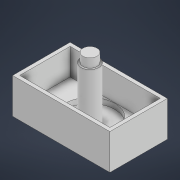
# Autodesk Inventor part: Servoverbindung_Konzept
Saved by Autodesk Inventor 2021 (Build 250183000, 183)
## iProperties
Created: 2021-01-13
Part Number: Servoverbindung_Konzept
Material: Generisch
Document SubType Name: Modeling
Designer: Ctroi
Density: 1 g/cm^3
Appearance: Vorgabe
Author: Ctroi
Autodesk Inventor part; units mm, degrees
ref_plane "YZ Plane" through (0, 0, 0) normal (1, 0, 0) x (0, 1, 0)
ref_plane "XZ Plane" through (0, 0, 0) normal (0, 1, 0) x (-1, 0, 0)
ref_plane "XY Plane" through (0, 0, 0) normal (0, 0, 1) x (1, 0, 0)
sketch "Skizze1" plane through (0, 0, 0) normal (0, 1, 0) x (-1, 0, 0)
  line L0 (-27.5, -16.25) -> (27.5, -16.25)
  line L1 (27.5, -16.25) -> (27.5, 16.25)
  line L2 (27.5, 16.25) -> (-27.5, 16.25)
  line L3 (-27.5, 16.25) -> (-27.5, -16.25)
  line L4 (-38.5, 0) -> (38.5, 0) projected
  line L5 (0, -22.75) -> (0, 22.75) projected
  point P0 (0, 0)
  dimension "d0" = 55
  dimension "d1" = 32.5
  constraints: 8 end point, 2 parallel, 1 horizontal, 1 perpendicular, 2 other
  measures "d0" distance of L1.end L2.end
  measures "d1" distance of L0.end L1.end
extrude "Extrusion1" add sketch "Skizze1" along normal blind 5
sketch "Skizze2" plane through (0, 5, 0) normal (0, 1, 0) x (1, 0, 0)
  circle A0 centre (0, 0) radius 14
  circle A1 centre (0, 0) radius 11
  dimension "d4" = 28
  dimension "d5" = 3
  constraints: 2 centre point, 1 coincident
  measures "d4" diameter of A0
  measures "d5" radial gap between concentric circles of A0 A1
extrude "Extrusion2" cut sketch "Skizze2" against normal blind 3 contours A0 | A1
sketch "Skizze3" plane through (0, 2, 0) normal (0, 1, 0) x (1, 0, 0)
  circle A0 centre (0, 0) radius 5
  dimension "d8" = 10
  constraints: 1 centre point, 1 coincident
  measures "d8" diameter of A0
extrude "Extrusion3" add sketch "Skizze3" along normal blind 30
sketch "Skizze4" plane through (0, 32, 0) normal (0, 1, 0) x (1, 0, 0)
  circle A0 centre (0, 0) radius 4
  dimension "d11" = 8
  constraints: 1 centre point, 1 coincident
  measures "d11" diameter of A0
extrude "Extrusion4" add sketch "Skizze4" along normal blind 5
sketch "Skizze5" plane through (0, 5, 0) normal (0, 1, 0) x (1, 0, 0)
  line L0 (27.5, 16.25) -> (-27.5, 16.25) projected
  line L1 (27.5, -16.25) -> (27.5, 16.25) projected
  line L2 (-27.5, 16.25) -> (27.5, 16.25)
  line L3 (27.5, 16.25) -> (27.5, -16.25)
  line L4 (27.5, -16.25) -> (-27.5, -16.25)
  line L5 (-27.5, -16.25) -> (-27.5, 16.25)
  line L6 (-25.5, 14.25) -> (25.5, 14.25)
  line L7 (25.5, 14.25) -> (25.5, -14.25)
  line L8 (25.5, -14.25) -> (-25.5, -14.25)
  line L9 (-25.5, -14.25) -> (-25.5, 14.25)
  point P0 (0, 0)
  dimension "d14" = 2
  constraints: 16 end point, 4 parallel, 2 perpendicular, 1 horizontal, 3 other
  measures "d14" distance between parallel lines of L5 L9
extrude "Extrusion5" add sketch "Skizze5" along normal blind 15
